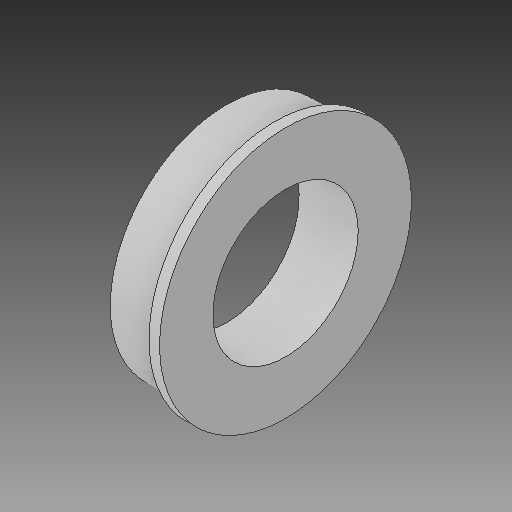
# Autodesk Inventor part: F6802
Saved by Autodesk Inventor 2019.4 (Build 234330000, 330)
## iProperties
Created: 2019-12-31
Part Number: F6802
Material: Generic
Document SubType Name: Modeling
Designer: Mark
Density: 1 g/cm^3
Appearance: Default
Mass: 1.76801 g
Surface Area: 14.6273 cm^2
Volume: 1.76801 cm^3
Author: Mark
Autodesk Inventor part; units mm, degrees
ref_plane "YZ Plane" through (0, 0, 0) normal (1, 0, 0) x (0, 1, 0)
ref_plane "XZ Plane" through (0, 0, 0) normal (0, 1, 0) x (-1, 0, 0)
ref_plane "XY Plane" through (0, 0, 0) normal (0, 0, 1) x (1, 0, 0)
sketch "Sketch1" plane through (0, 0, 0) normal (1, 0, 0) x (0, 1, 0)
  circle A0 centre (0, 0) radius 12
  circle A1 centre (0, 0) radius 7.5
  dimension "d0" = 24
  dimension "d1" = 15
  constraints: 2 centre point, 2 coincident
  measures "d0" diameter of A0
  measures "d1" diameter of A1
extrude "Extrusion1" add sketch "Sketch1" along normal blind 5
sketch "Sketch2" plane through (5, 0, 0) normal (1, 0, 0) x (0, 0, -1)
  circle A0 centre (0, 0) radius 7.5
  circle A1 centre (0, 0) radius 13
  dimension "d4" = 15
  dimension "d5" = 26
  constraints: 2 centre point, 2 coincident
  measures "d4" diameter of A0
  measures "d5" diameter of A1
extrude "Extrusion2" add sketch "Sketch2" along normal blind 1.1
body "Solid1"
